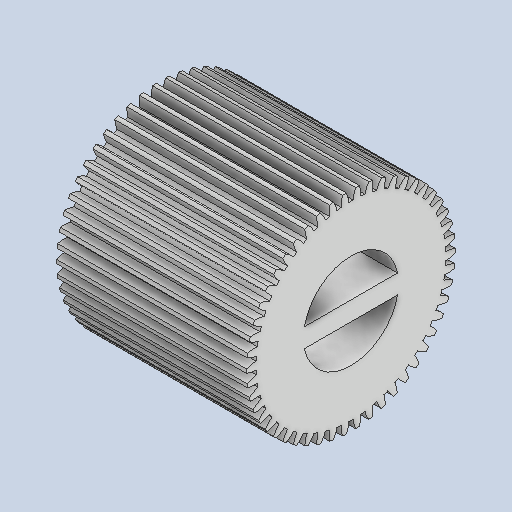
# Autodesk Inventor part: 평기어_가변저항
Saved by Autodesk Inventor 2024 (Build 280153000, 153)
## iProperties
Created: 2024-04-20
Part Number: 평기어_가변저항
Material: 일반
Document SubType Name: Modeling
Designer: kkamin5
Density: 1 g/cm^3
Appearance: 기본값
Author: kkamin5
Autodesk Inventor part; units mm, degrees
ref_plane "YZ Plane" through (0, 0, 0) normal (1, 0, 0) x (0, 1, 0)
ref_plane "XZ Plane" through (0, 0, 0) normal (0, 1, 0) x (-1, 0, 0)
ref_plane "XY Plane" through (0, 0, 0) normal (0, 0, 1) x (1, 0, 0)
sketch "스케치1" plane through (0, 0, 0) normal (1, 0, 0) x (0, 1, 0)
  line L0 (0, -5.5) -> (0.1, -5.5)
  arc A0 (0.1, -5.5) -> (0.2033, -4.8791) centre (-1.3293, -4.9431) ccw
  line L1 (0, 0) -> (0, -6.6238) construction
  line L2 (0, -5.5) -> (-0.1, -5.5)
  arc A1 (-0.2033, -4.8791) -> (-0.1, -5.5) centre (1.3293, -4.9431) ccw
  line L3 (0.6893, -5.4566) -> (0.7885, -5.4441)
  arc A2 (0.7885, -5.4441) -> (0.8132, -4.8151) centre (-0.6993, -5.0708) ccw
  line L4 (0, 0) -> (0.8302, -6.5716) construction
  line L5 (0.6893, -5.4566) -> (0.5901, -5.4692)
  arc A3 (0.4098, -4.8661) -> (0.5901, -5.4692) centre (1.9383, -4.7375) ccw
  line L6 (1.3678, -5.3272) -> (1.4647, -5.3023)
  arc A4 (1.4647, -5.3023) -> (1.4103, -4.6752) centre (-0.0582, -5.1184) ccw
  line L7 (0, 0) -> (1.6473, -6.4157) construction
  line L8 (1.3678, -5.3272) -> (1.2709, -5.3521)
  arc A5 (1.0165, -4.7764) -> (1.2709, -5.3521) centre (2.5168, -4.4572) ccw
  line L9 (2.0247, -5.1138) -> (2.1177, -5.077)
  arc A6 (2.1177, -5.077) -> (1.9851, -4.4616) centre (0.5837, -5.0853) ccw
  line L10 (0, 0) -> (2.4384, -6.1586) construction
  line L11 (2.0247, -5.1138) -> (1.9317, -5.1506)
  arc A7 (1.6071, -4.6113) -> (1.9317, -5.1506) centre (3.0556, -4.1067) ccw
  line L12 (2.6496, -4.8197) -> (2.7373, -4.7715)
  arc A8 (2.7373, -4.7715) -> (2.5287, -4.1776) centre (1.2165, -4.9721) ccw
  line L13 (0, 0) -> (3.191, -5.8045) construction
  line L14 (2.6496, -4.8197) -> (2.562, -4.8679)
  arc A9 (2.1724, -4.3735) -> (2.562, -4.8679) centre (3.5462, -3.6913) ccw
  line L15 (3.2328, -4.4496) -> (3.3137, -4.3908)
  arc A10 (3.3137, -4.3908) -> (3.0323, -3.8278) centre (1.8301, -4.7804) ccw
  line L16 (0, 0) -> (3.8934, -5.3588) construction
  line L17 (3.2328, -4.4496) -> (3.1519, -4.5084)
  arc A11 (2.7034, -4.0668) -> (3.1519, -4.5084) centre (3.9809, -3.2177) ccw
  line L18 (3.765, -4.0093) -> (3.8379, -3.9409)
  arc A12 (3.8379, -3.9409) -> (3.4882, -3.4175) centre (2.4148, -4.5133) ccw
  line L19 (0, 0) -> (4.5343, -4.8285) construction
  line L20 (3.765, -4.0093) -> (3.6921, -4.0778)
  arc A13 (3.1918, -3.6959) -> (3.6921, -4.0778) centre (4.3528, -2.6934) ccw
  line L21 (4.2378, -3.5058) -> (4.3016, -3.4288)
  arc A14 (4.3016, -3.4288) -> (3.889, -2.9534) centre (2.9614, -4.1751) ccw
  line L22 (0, 0) -> (5.1037, -4.2222) construction
  line L23 (4.2378, -3.5058) -> (4.1741, -3.5829)
  arc A15 (3.6298, -3.2667) -> (4.1741, -3.5829) centre (4.6561, -2.1266) ccw
  line L24 (4.6438, -2.947) -> (4.6974, -2.8626)
  arc A16 (4.6974, -2.8626) -> (4.2285, -2.4427) centre (3.4614, -3.771) ccw
  line L25 (0, 0) -> (5.5927, -3.5492) construction
  line L26 (4.6438, -2.947) -> (4.5902, -3.0315)
  arc A17 (4.0106, -2.786) -> (4.5902, -3.0315) centre (4.8859, -1.5263) ccw
  line L27 (4.9765, -2.3418) -> (5.0191, -2.2513)
  arc A18 (5.0191, -2.2513) -> (4.5013, -1.8934) centre (3.9067, -3.3075) ccw
  line L28 (0, 0) -> (5.9934, -2.8203) construction
  line L29 (4.9765, -2.3418) -> (4.934, -2.4323)
  arc A19 (4.3282, -2.2614) -> (4.934, -2.4323) centre (5.0387, -0.9019) ccw
  line L30 (5.2308, -1.6996) -> (5.2617, -1.6045)
  arc A20 (5.2617, -1.6045) -> (4.7031, -1.3144) centre (4.2904, -2.7917) ccw
  line L31 (0, 0) -> (6.2996, -2.0469) construction
  line L32 (5.2308, -1.6996) -> (5.1999, -1.7947)
  arc A21 (4.5775, -1.7011) -> (5.1999, -1.7947) centre (5.112, -0.2633) ccw
  line L33 (5.4026, -1.0306) -> (5.4213, -0.9324)
  arc A22 (5.4213, -0.9324) -> (4.8308, -0.7145) centre (4.6065, -2.232) ccw
  line L34 (0, 0) -> (6.5065, -1.2412) construction
  line L35 (5.4026, -1.0306) -> (5.3838, -1.1288)
  arc A23 (4.7546, -1.114) -> (5.3838, -1.1288) centre (5.1047, 0.3795) ccw
  line L36 (5.4891, -0.3453) -> (5.4954, -0.2455)
  arc A24 (5.4954, -0.2455) -> (4.8822, -0.1034) centre (4.8499, -1.637) ccw
  line L37 (0, 0) -> (6.6107, -0.4159) construction
  line L38 (5.4891, -0.3453) -> (5.4829, -0.4452)
  arc A25 (4.8567, -0.5093) -> (5.4829, -0.4452) centre (5.0168, 1.0163) ccw
  line L39 (5.4891, 0.3453) -> (5.4829, 0.4452)
  arc A26 (5.4829, 0.4452) -> (4.8567, 0.5093) centre (5.0168, -1.0163) ccw
  line L40 (0, 0) -> (6.6107, 0.4159) construction
  line L41 (5.4891, 0.3453) -> (5.4954, 0.2455)
  arc A27 (4.8822, 0.1034) -> (5.4954, 0.2455) centre (4.8499, 1.637) ccw
  line L42 (5.4026, 1.0306) -> (5.3838, 1.1288)
  arc A28 (5.3838, 1.1288) -> (4.7546, 1.114) centre (5.1047, -0.3795) ccw
  line L43 (0, 0) -> (6.5065, 1.2412) construction
  line L44 (5.4026, 1.0306) -> (5.4213, 0.9324)
  arc A29 (4.8308, 0.7145) -> (5.4213, 0.9324) centre (4.6065, 2.232) ccw
  line L45 (5.2308, 1.6996) -> (5.1999, 1.7947)
  arc A30 (5.1999, 1.7947) -> (4.5775, 1.7011) centre (5.112, 0.2633) ccw
  line L46 (0, 0) -> (6.2996, 2.0469) construction
  line L47 (5.2308, 1.6996) -> (5.2617, 1.6045)
  arc A31 (4.7031, 1.3144) -> (5.2617, 1.6045) centre (4.2904, 2.7917) ccw
  line L48 (4.9765, 2.3418) -> (4.934, 2.4323)
  arc A32 (4.934, 2.4323) -> (4.3282, 2.2614) centre (5.0387, 0.9019) ccw
  line L49 (0, 0) -> (5.9934, 2.8203) construction
  line L50 (4.9765, 2.3418) -> (5.0191, 2.2513)
  arc A33 (4.5013, 1.8934) -> (5.0191, 2.2513) centre (3.9067, 3.3075) ccw
  line L51 (4.6438, 2.947) -> (4.5902, 3.0315)
  arc A34 (4.5902, 3.0315) -> (4.0106, 2.786) centre (4.8859, 1.5263) ccw
  line L52 (0, 0) -> (5.5927, 3.5492) construction
  line L53 (4.6438, 2.947) -> (4.6974, 2.8626)
  arc A35 (4.2285, 2.4427) -> (4.6974, 2.8626) centre (3.4614, 3.771) ccw
  line L54 (4.2378, 3.5058) -> (4.1741, 3.5829)
  arc A36 (4.1741, 3.5829) -> (3.6298, 3.2667) centre (4.6561, 2.1266) ccw
  line L55 (0, 0) -> (5.1037, 4.2222) construction
  line L56 (4.2378, 3.5058) -> (4.3016, 3.4288)
  arc A37 (3.889, 2.9534) -> (4.3016, 3.4288) centre (2.9614, 4.1751) ccw
  line L57 (3.765, 4.0093) -> (3.6921, 4.0778)
  arc A38 (3.6921, 4.0778) -> (3.1918, 3.6959) centre (4.3528, 2.6934) ccw
  line L58 (0, 0) -> (4.5343, 4.8285) construction
  line L59 (3.765, 4.0093) -> (3.8379, 3.9409)
  arc A39 (3.4882, 3.4175) -> (3.8379, 3.9409) centre (2.4148, 4.5133) ccw
  line L60 (3.2328, 4.4496) -> (3.1519, 4.5084)
  arc A40 (3.1519, 4.5084) -> (2.7034, 4.0668) centre (3.9809, 3.2177) ccw
  line L61 (0, 0) -> (3.8934, 5.3588) construction
  line L62 (3.2328, 4.4496) -> (3.3137, 4.3908)
  arc A41 (3.0323, 3.8278) -> (3.3137, 4.3908) centre (1.8301, 4.7804) ccw
  line L63 (2.6496, 4.8197) -> (2.562, 4.8679)
  arc A42 (2.562, 4.8679) -> (2.1724, 4.3735) centre (3.5462, 3.6913) ccw
  line L64 (0, 0) -> (3.191, 5.8045) construction
  line L65 (2.6496, 4.8197) -> (2.7373, 4.7715)
  arc A43 (2.5287, 4.1776) -> (2.7373, 4.7715) centre (1.2165, 4.9721) ccw
  line L66 (2.0247, 5.1138) -> (1.9317, 5.1506)
  arc A44 (1.9317, 5.1506) -> (1.6071, 4.6113) centre (3.0556, 4.1067) ccw
  line L67 (0, 0) -> (2.4384, 6.1586) construction
  line L68 (2.0247, 5.1138) -> (2.1177, 5.077)
  arc A45 (1.9851, 4.4616) -> (2.1177, 5.077) centre (0.5837, 5.0853) ccw
  line L69 (1.3678, 5.3272) -> (1.2709, 5.3521)
  arc A46 (1.2709, 5.3521) -> (1.0165, 4.7764) centre (2.5168, 4.4572) ccw
  line L70 (0, 0) -> (1.6473, 6.4157) construction
  line L71 (1.3678, 5.3272) -> (1.4647, 5.3023)
  arc A47 (1.4103, 4.6752) -> (1.4647, 5.3023) centre (-0.0582, 5.1184) ccw
  line L72 (0.6893, 5.4566) -> (0.5901, 5.4692)
  arc A48 (0.5901, 5.4692) -> (0.4098, 4.8661) centre (1.9383, 4.7375) ccw
  line L73 (0, 0) -> (0.8302, 6.5716) construction
  line L74 (0.6893, 5.4566) -> (0.7885, 5.4441)
  arc A49 (0.8132, 4.8151) -> (0.7885, 5.4441) centre (-0.6993, 5.0708) ccw
  line L75 (0, 5.5) -> (-0.1, 5.5)
  arc A50 (-0.1, 5.5) -> (-0.2033, 4.8791) centre (1.3293, 4.9431) ccw
  line L76 (0, 0) -> (0, 6.6238) construction
  line L77 (0, 5.5) -> (0.1, 5.5)
  arc A51 (0.2033, 4.8791) -> (0.1, 5.5) centre (-1.3293, 4.9431) ccw
  line L78 (-0.6893, 5.4566) -> (-0.7885, 5.4441)
  arc A52 (-0.7885, 5.4441) -> (-0.8132, 4.8151) centre (0.6993, 5.0708) ccw
  line L79 (0, 0) -> (-0.8302, 6.5716) construction
  line L80 (-0.6893, 5.4566) -> (-0.5901, 5.4692)
  arc A53 (-0.4098, 4.8661) -> (-0.5901, 5.4692) centre (-1.9383, 4.7375) ccw
  line L81 (-1.3678, 5.3272) -> (-1.4647, 5.3023)
  arc A54 (-1.4647, 5.3023) -> (-1.4103, 4.6752) centre (0.0582, 5.1184) ccw
  line L82 (0, 0) -> (-1.6473, 6.4157) construction
  line L83 (-1.3678, 5.3272) -> (-1.2709, 5.3521)
  arc A55 (-1.0165, 4.7764) -> (-1.2709, 5.3521) centre (-2.5168, 4.4572) ccw
  line L84 (-2.0247, 5.1138) -> (-2.1177, 5.077)
  arc A56 (-2.1177, 5.077) -> (-1.9851, 4.4616) centre (-0.5837, 5.0853) ccw
  line L85 (0, 0) -> (-2.4384, 6.1586) construction
  line L86 (-2.0247, 5.1138) -> (-1.9317, 5.1506)
  arc A57 (-1.6071, 4.6113) -> (-1.9317, 5.1506) centre (-3.0556, 4.1067) ccw
  line L87 (-2.6496, 4.8197) -> (-2.7373, 4.7715)
  arc A58 (-2.7373, 4.7715) -> (-2.5287, 4.1776) centre (-1.2165, 4.9721) ccw
  line L88 (0, 0) -> (-3.191, 5.8045) construction
  line L89 (-2.6496, 4.8197) -> (-2.562, 4.8679)
  arc A59 (-2.1724, 4.3735) -> (-2.562, 4.8679) centre (-3.5462, 3.6913) ccw
  line L90 (-3.2328, 4.4496) -> (-3.3137, 4.3908)
  arc A60 (-3.3137, 4.3908) -> (-3.0323, 3.8278) centre (-1.8301, 4.7804) ccw
  line L91 (0, 0) -> (-3.8934, 5.3588) construction
  line L92 (-3.2328, 4.4496) -> (-3.1519, 4.5084)
  arc A61 (-2.7034, 4.0668) -> (-3.1519, 4.5084) centre (-3.9809, 3.2177) ccw
  line L93 (-3.765, 4.0093) -> (-3.8379, 3.9409)
  arc A62 (-3.8379, 3.9409) -> (-3.4882, 3.4175) centre (-2.4148, 4.5133) ccw
  line L94 (0, 0) -> (-4.5343, 4.8285) construction
  line L95 (-3.765, 4.0093) -> (-3.6921, 4.0778)
  arc A63 (-3.1918, 3.6959) -> (-3.6921, 4.0778) centre (-4.3528, 2.6934) ccw
  line L96 (-4.2378, 3.5058) -> (-4.3016, 3.4288)
  arc A64 (-4.3016, 3.4288) -> (-3.889, 2.9534) centre (-2.9614, 4.1751) ccw
  line L97 (0, 0) -> (-5.1037, 4.2222) construction
  line L98 (-4.2378, 3.5058) -> (-4.1741, 3.5829)
  arc A65 (-3.6298, 3.2667) -> (-4.1741, 3.5829) centre (-4.6561, 2.1266) ccw
  line L99 (-4.6438, 2.947) -> (-4.6974, 2.8626)
  arc A66 (-4.6974, 2.8626) -> (-4.2285, 2.4427) centre (-3.4614, 3.771) ccw
  line L100 (0, 0) -> (-5.5927, 3.5492) construction
  line L101 (-4.6438, 2.947) -> (-4.5902, 3.0315)
  arc A67 (-4.0106, 2.786) -> (-4.5902, 3.0315) centre (-4.8859, 1.5263) ccw
  line L102 (-4.9765, 2.3418) -> (-5.0191, 2.2513)
  arc A68 (-5.0191, 2.2513) -> (-4.5013, 1.8934) centre (-3.9067, 3.3075) ccw
  line L103 (0, 0) -> (-5.9934, 2.8203) construction
  line L104 (-4.9765, 2.3418) -> (-4.934, 2.4323)
  arc A69 (-4.3282, 2.2614) -> (-4.934, 2.4323) centre (-5.0387, 0.9019) ccw
  line L105 (-5.2308, 1.6996) -> (-5.2617, 1.6045)
  arc A70 (-5.2617, 1.6045) -> (-4.7031, 1.3144) centre (-4.2904, 2.7917) ccw
  line L106 (0, 0) -> (-6.2996, 2.0469) construction
  line L107 (-5.2308, 1.6996) -> (-5.1999, 1.7947)
  arc A71 (-4.5775, 1.7011) -> (-5.1999, 1.7947) centre (-5.112, 0.2633) ccw
  line L108 (-5.4026, 1.0306) -> (-5.4213, 0.9324)
  arc A72 (-5.4213, 0.9324) -> (-4.8308, 0.7145) centre (-4.6065, 2.232) ccw
  line L109 (0, 0) -> (-6.5065, 1.2412) construction
  line L110 (-5.4026, 1.0306) -> (-5.3838, 1.1288)
  arc A73 (-4.7546, 1.114) -> (-5.3838, 1.1288) centre (-5.1047, -0.3795) ccw
  line L111 (-5.4891, 0.3453) -> (-5.4954, 0.2455)
  arc A74 (-5.4954, 0.2455) -> (-4.8822, 0.1034) centre (-4.8499, 1.637) ccw
  line L112 (0, 0) -> (-6.6107, 0.4159) construction
  line L113 (-5.4891, 0.3453) -> (-5.4829, 0.4452)
  arc A75 (-4.8567, 0.5093) -> (-5.4829, 0.4452) centre (-5.0168, -1.0163) ccw
  line L114 (-5.4891, -0.3453) -> (-5.4829, -0.4452)
  arc A76 (-5.4829, -0.4452) -> (-4.8567, -0.5093) centre (-5.0168, 1.0163) ccw
  line L115 (0, 0) -> (-6.6107, -0.4159) construction
  line L116 (-5.4891, -0.3453) -> (-5.4954, -0.2455)
  arc A77 (-4.8822, -0.1034) -> (-5.4954, -0.2455) centre (-4.8499, -1.637) ccw
  line L117 (-5.4026, -1.0306) -> (-5.3838, -1.1288)
  arc A78 (-5.3838, -1.1288) -> (-4.7546, -1.114) centre (-5.1047, 0.3795) ccw
  line L118 (0, 0) -> (-6.5065, -1.2412) construction
  line L119 (-5.4026, -1.0306) -> (-5.4213, -0.9324)
  arc A79 (-4.8308, -0.7145) -> (-5.4213, -0.9324) centre (-4.6065, -2.232) ccw
  line L120 (-5.2308, -1.6996) -> (-5.1999, -1.7947)
  arc A80 (-5.1999, -1.7947) -> (-4.5775, -1.7011) centre (-5.112, -0.2633) ccw
  line L121 (0, 0) -> (-6.2996, -2.0469) construction
  line L122 (-5.2308, -1.6996) -> (-5.2617, -1.6045)
  arc A81 (-4.7031, -1.3144) -> (-5.2617, -1.6045) centre (-4.2904, -2.7917) ccw
  line L123 (-4.9765, -2.3418) -> (-4.934, -2.4323)
  arc A82 (-4.934, -2.4323) -> (-4.3282, -2.2614) centre (-5.0387, -0.9019) ccw
  line L124 (0, 0) -> (-5.9934, -2.8203) construction
  line L125 (-4.9765, -2.3418) -> (-5.0191, -2.2513)
  arc A83 (-4.5013, -1.8934) -> (-5.0191, -2.2513) centre (-3.9067, -3.3075) ccw
  line L126 (-4.6438, -2.947) -> (-4.5902, -3.0315)
  arc A84 (-4.5902, -3.0315) -> (-4.0106, -2.786) centre (-4.8859, -1.5263) ccw
  line L127 (0, 0) -> (-5.5927, -3.5492) construction
  line L128 (-4.6438, -2.947) -> (-4.6974, -2.8626)
  arc A85 (-4.2285, -2.4427) -> (-4.6974, -2.8626) centre (-3.4614, -3.771) ccw
  line L129 (-4.2378, -3.5058) -> (-4.1741, -3.5829)
  arc A86 (-4.1741, -3.5829) -> (-3.6298, -3.2667) centre (-4.6561, -2.1266) ccw
  line L130 (0, 0) -> (-5.1037, -4.2222) construction
  line L131 (-4.2378, -3.5058) -> (-4.3016, -3.4288)
  arc A87 (-3.889, -2.9534) -> (-4.3016, -3.4288) centre (-2.9614, -4.1751) ccw
  line L132 (-3.765, -4.0093) -> (-3.6921, -4.0778)
  arc A88 (-3.6921, -4.0778) -> (-3.1918, -3.6959) centre (-4.3528, -2.6934) ccw
  line L133 (0, 0) -> (-4.5343, -4.8285) construction
  line L134 (-3.765, -4.0093) -> (-3.8379, -3.9409)
  arc A89 (-3.4882, -3.4175) -> (-3.8379, -3.9409) centre (-2.4148, -4.5133) ccw
  line L135 (-3.2328, -4.4496) -> (-3.1519, -4.5084)
  arc A90 (-3.1519, -4.5084) -> (-2.7034, -4.0668) centre (-3.9809, -3.2177) ccw
  line L136 (0, 0) -> (-3.8934, -5.3588) construction
  line L137 (-3.2328, -4.4496) -> (-3.3137, -4.3908)
  arc A91 (-3.0323, -3.8278) -> (-3.3137, -4.3908) centre (-1.8301, -4.7804) ccw
  line L138 (-2.6496, -4.8197) -> (-2.562, -4.8679)
  arc A92 (-2.562, -4.8679) -> (-2.1724, -4.3735) centre (-3.5462, -3.6913) ccw
  line L139 (0, 0) -> (-3.191, -5.8045) construction
  line L140 (-2.6496, -4.8197) -> (-2.7373, -4.7715)
  arc A93 (-2.5287, -4.1776) -> (-2.7373, -4.7715) centre (-1.2165, -4.9721) ccw
  line L141 (-2.0247, -5.1138) -> (-1.9317, -5.1506)
  arc A94 (-1.9317, -5.1506) -> (-1.6071, -4.6113) centre (-3.0556, -4.1067) ccw
  line L142 (0, 0) -> (-2.4384, -6.1586) construction
  line L143 (-2.0247, -5.1138) -> (-2.1177, -5.077)
  arc A95 (-1.9851, -4.4616) -> (-2.1177, -5.077) centre (-0.5837, -5.0853) ccw
  line L144 (-1.3678, -5.3272) -> (-1.2709, -5.3521)
  arc A96 (-1.2709, -5.3521) -> (-1.0165, -4.7764) centre (-2.5168, -4.4572) ccw
  line L145 (0, 0) -> (-1.6473, -6.4157) construction
  line L146 (-1.3678, -5.3272) -> (-1.4647, -5.3023)
  arc A97 (-1.4103, -4.6752) -> (-1.4647, -5.3023) centre (0.0582, -5.1184) ccw
  line L147 (-0.6893, -5.4566) -> (-0.5901, -5.4692)
  arc A98 (-0.5901, -5.4692) -> (-0.4098, -4.8661) centre (-1.9383, -4.7375) ccw
  line L148 (0, 0) -> (-0.8302, -6.5716) construction
  line L149 (-0.6893, -5.4566) -> (-0.7885, -5.4441)
  arc A99 (-0.8132, -4.8151) -> (-0.7885, -5.4441) centre (0.6993, -5.0708) ccw
  line L150 (5, 0) -> (50, 0)
  arc A100 (-5, 0) -> (5, 0) centre (0, 0) ccw
  circle A101 centre (0, 0) radius 5
  point P0 (0, -5)
  point P1 (4.9732, 0.517)
  point P2 (4.9455, 0.736)
  point P3 (4.8692, 1.1363)
  point P4 (4.8143, 1.35)
  point P5 (4.6884, 1.7376)
  point P6 (4.6071, 1.9428)
  point P7 (4.4336, 2.3115)
  point P8 (4.3273, 2.5049)
  point P9 (4.109, 2.8489)
  point P10 (3.9792, 3.0275)
  point P11 (3.7195, 3.3415)
  point P12 (3.5684, 3.5023)
  point P13 (3.2714, 3.7813)
  point P14 (3.1013, 3.922)
  point P15 (2.7717, 4.1615)
  point P16 (2.5853, 4.2797)
  point P17 (2.2282, 4.476)
  point P18 (2.0285, 4.57)
  point P19 (1.6497, 4.72)
  point P20 (1.4398, 4.7882)
  point P21 (1.0451, 4.8896)
  point P22 (0.8283, 4.9309)
  point P23 (0.424, 4.982)
  point P24 (0.2037, 4.9958)
  point P25 (-0.2037, 4.9958)
  point P26 (-0.424, 4.982)
  point P27 (-0.8283, 4.9309)
  point P28 (-1.0451, 4.8896)
  point P29 (-1.4398, 4.7882)
  point P30 (-1.6497, 4.72)
  point P31 (-2.0285, 4.57)
  point P32 (-2.2282, 4.476)
  point P33 (-2.5853, 4.2797)
  point P34 (-2.7717, 4.1615)
  point P35 (-3.1013, 3.922)
  point P36 (-3.2714, 3.7813)
  point P37 (-3.5684, 3.5023)
  point P38 (-3.7195, 3.3415)
  point P39 (-3.9792, 3.0275)
  point P40 (-4.109, 2.8489)
  point P41 (-4.3273, 2.5049)
  point P42 (-4.4336, 2.3115)
  point P43 (-4.6071, 1.9428)
  point P44 (-4.6884, 1.7376)
  point P45 (-4.8143, 1.35)
  point P46 (-4.8692, 1.1363)
  point P47 (-4.9455, 0.736)
  point P48 (-4.9732, 0.517)
  point P49 (-4.9988, 0.1103)
  point P50 (-4.9988, -0.1103)
  point P51 (-4.9732, -0.517)
  point P52 (-4.9455, -0.736)
  point P53 (-4.8692, -1.1363)
  point P54 (-4.8143, -1.35)
  point P55 (-4.6884, -1.7376)
  point P56 (-4.6071, -1.9428)
  point P57 (-4.4336, -2.3115)
  point P58 (-4.3273, -2.5049)
  point P59 (-4.109, -2.8489)
  point P60 (-3.9792, -3.0275)
  point P61 (-3.7195, -3.3415)
  point P62 (-3.5684, -3.5023)
  point P63 (-3.2714, -3.7813)
  point P64 (-3.1013, -3.922)
  point P65 (-2.7717, -4.1615)
  point P66 (-2.5853, -4.2797)
  point P67 (-2.2282, -4.476)
  point P68 (-2.0285, -4.57)
  point P69 (-1.6497, -4.72)
  point P70 (-1.4398, -4.7882)
  point P71 (-1.0451, -4.8896)
  point P72 (-0.8283, -4.9309)
  point P73 (-0.424, -4.982)
  point P74 (-0.2037, -4.9958)
  point P75 (0.2037, -4.9958)
  point P76 (0.424, -4.982)
  point P77 (0.8283, -4.9309)
  point P78 (1.0451, -4.8896)
  point P79 (1.4398, -4.7882)
  point P80 (1.6497, -4.72)
  point P81 (2.0285, -4.57)
  point P82 (2.2282, -4.476)
  point P83 (2.5853, -4.2797)
  point P84 (2.7717, -4.1615)
  point P85 (3.1013, -3.922)
  point P86 (3.2714, -3.7813)
  point P87 (3.5684, -3.5023)
  point P88 (3.7195, -3.3415)
  point P89 (3.9792, -3.0275)
  point P90 (4.109, -2.8489)
  point P91 (4.3273, -2.5049)
  point P92 (4.4336, -2.3115)
  point P93 (4.6071, -1.9428)
  point P94 (4.6884, -1.7376)
  point P95 (4.8143, -1.35)
  point P96 (4.8692, -1.1363)
  point P97 (4.9455, -0.736)
  point P98 (4.9732, -0.517)
  point P99 (4.9988, -0.1103)
  point P100 (5, 0)
  point P101 (4.9988, 0.1103)
  dimension "d2" = 360
  dimension "d3" = 0.5
  constraints: 302 end point, 200 point on circle, 100 centre point, 4 coincident, 3 symmetric about line, 1 horizontal, 1 vertical, 713 other
  measures "d3" distance from line of L0 point (0, -5)
extrude "돌출1" add sketch "스케치1" along normal mid plane 10
sketch "스케치2" plane through (5, 0, 0) normal (1, 0, 0) x (0, 0, -1)
  circle A0 centre (0, 0) radius 2.5
  dimension "d6" = 5
  constraints: 1 centre point, 1 coincident
  measures "d6" diameter of A0
extrude "돌출2" cut sketch "스케치2" against normal blind 10
sketch "스케치3" plane through (5, 0, 0) normal (1, 0, 0) x (0, 0, -1)
  line L0 (-3.5512, 0.5) -> (4.0111, 0.5)
  line L1 (4.0111, 0.5) -> (4.0111, -0.5)
  line L2 (4.0111, -0.5) -> (-3.5512, -0.5)
  line L3 (-3.5512, -0.5) -> (-3.5512, 0.5)
  point P0 (0, 0)
  dimension "d9" = 1
  dimension "d10" = 0.5
  constraints: 8 end point, 2 parallel, 1 horizontal, 1 perpendicular
  measures "d9" distance of L0.end L1.end
  measures "d10" distance from line of point (0, 0) L2
extrude "돌출3" add sketch "스케치3" against normal blind 10
equation "\"d10\" = 0.5 * d9"
